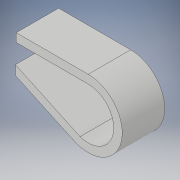
# Autodesk Inventor part: 01_Laser_Clamp_OnOffSwitch
Saved by Autodesk Inventor 2019 (Build 230136000, 136)
## iProperties
Created: 2019-05-07
Part Number: 01_Laser_Clamp_OnOffSwitch
Material: Generic
Document SubType Name: Modeling
Designer: diederichbenedict
Density: 1 g/cm^3
Appearance: Default
Author: diederichbenedict
Autodesk Inventor part; units mm, degrees
ref_plane "YZ Plane" through (0, 0, 0) normal (1, 0, 0) x (0, 1, 0)
ref_plane "XZ Plane" through (0, 0, 0) normal (0, 1, 0) x (-1, 0, 0)
ref_plane "XY Plane" through (0, 0, 0) normal (0, 0, 1) x (1, 0, 0)
sketch "Sketch1" plane through (0, 0, 0) normal (0, 0, 1) x (1, 0, 0)
  circle A0 centre (-0.2626, 0.8226) radius 5.775
  line L0 (-5.743, 8.5976) -> (11.2384, 8.5976)
  arc A1 (8.5691, -6.944) -> (11.2384, 8.5976) centre (11.2384, 0.5976) ccw
  line L1 (8.5691, -6.944) -> (-5.9413, -0.2275)
  line L2 (-5.743, 6.5976) -> (11.2384, 6.5976)
  arc A2 (9.3184, -5.0869) -> (11.2384, 6.5976) centre (11.2384, 0.5976) ccw
  line L3 (9.3184, -5.0869) -> (-5.9413, 1.9763)
  line L4 (-5.743, 8.5976) -> (-5.743, 6.5976)
  line L5 (-5.9413, 1.9763) -> (-5.9413, -0.2275)
  point P0 (0, 0)
  dimension "d6" = 11.55
  dimension "d0" = 6
  dimension "d2" = 2
  dimension "d3" = 90
  constraints: 12 end point, 4 point on circle, 2 centre point, 2 horizontal, 1 parallel, 1 tangent, 5 other
  measures "d0" radius of A2
  measures "d2" distance between parallel lines of L2 L0
  measures "d3" angle of L0 L4
extrude "Extrusion1" add sketch "Sketch1" along normal blind 10 contours L2 L4 L0 A1 L1 A0 L3 A2 | A0 L1 L5 L3 | A0 L5 L3
body "Solid1"
